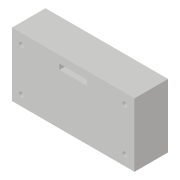
# Autodesk Inventor part: Display
Saved by Autodesk Inventor 2018 (Build 220112000, 112)
## iProperties
Created: 2019-01-22
Part Number: Display
Material: Generic
Document SubType Name: Modeling
Designer: ball
Density: 1 g/cm^3
Appearance: Default
Author: ball
Autodesk Inventor part; units mm, degrees
ref_plane "YZ Plane" through (0, 0, 0) normal (1, 0, 0) x (0, 1, 0)
ref_plane "XZ Plane" through (0, 0, 0) normal (0, 1, 0) x (-1, 0, 0)
sketch "Sketch1" plane through (0, 0, 0) normal (0, 0, 1) x (1, 0, 0)
  line L0 (-27.559, -14.2875) -> (27.559, -14.2875)
  line L1 (27.559, -14.2875) -> (27.559, 14.2875)
  line L2 (27.559, 14.2875) -> (-27.559, 14.2875)
  line L3 (-27.559, 14.2875) -> (-27.559, -14.2875)
  line L4 (-27.559, -14.2875) -> (27.559, 14.2875) construction
  line L5 (27.559, -14.2875) -> (-27.559, 14.2875) construction
  line L6 (0, 0) -> (0, 51.7616) construction
  line L7 (-6.223, 8.4963) -> (6.223, 8.4963)
  line L8 (6.223, 8.4963) -> (6.223, 10.9347)
  line L9 (6.223, 10.9347) -> (-6.223, 10.9347)
  line L10 (-6.223, 10.9347) -> (-6.223, 8.4963)
  line L11 (-6.223, 8.4963) -> (6.223, 10.9347) construction
  line L12 (6.223, 8.4963) -> (-6.223, 10.9347) construction
  circle A0 centre (-23.241, 9.7155) radius 1.0795
  circle A1 centre (23.241, 9.7155) radius 1.0795
  circle A2 centre (-23.241, -9.7155) radius 1.0795
  circle A3 centre (23.241, -9.7155) radius 1.0795
  point P0 (0, 9.7155)
  dimension "d0" = 55.118
  dimension "d1" = 28.575
  dimension "d2" = 12.446
  dimension "d3" = 2.4384
  dimension "d11" = 4.572
  dimension "d12" = 2.159
  dimension "d13" = 2.159
  dimension "d14" = 4.318
  dimension "d15" = 4.318
  dimension "d16" = 2.159
  dimension "d17" = 4.572
  dimension "d18" = 2.159
  constraints: 26 end point, 4 centre point, 4 midpoint, 4 parallel, 2 horizontal, 2 perpendicular, 1 point on line, 1 vertical
  measures "d0" distance of L1.end L2.end
  measures "d1" distance of L0.end L1.end
  measures "d2" distance of L8.end L9.end
  measures "d3" distance of L9.end L7.start
  measures "d11" distance from line of L2 point (0, 9.715)
  measures "d12" diameter of A0
  measures "d13" diameter of A1
  measures "d14" distance from line of L3 A0.centre
  measures "d15" distance from line of L1 A1.centre
  measures "d16" diameter of A2
  measures "d17" distance from line of L0 A2.centre
  measures "d18" diameter of A3
ref_plane "Work Plane1" through (0, 0, 11.938) normal (0, 0, 1) x (1, 0, 0)
sketch "Sketch2" plane through (0, 0, 11.938) normal (0, 0, 1) x (1, 0, 0)
  line L0 (-25.019, -11.7475) -> (25.019, -11.7475)
  line L1 (25.019, -11.7475) -> (25.019, 11.7475)
  line L2 (25.019, 11.7475) -> (-25.019, 11.7475)
  line L3 (-25.019, 11.7475) -> (-25.019, -11.7475)
  line L4 (-25.019, -11.7475) -> (25.019, 11.7475) construction
  line L5 (25.019, -11.7475) -> (-25.019, 11.7475) construction
  line L6 (27.559, 14.2875) -> (-27.559, 14.2875) projected
  line L7 (-27.559, 14.2875) -> (-27.559, -14.2875) projected
  point P0 (0, 0)
  dimension "d7" = 2.54
  dimension "d8" = 2.54
  constraints: 12 end point, 2 midpoint, 2 parallel, 1 horizontal, 1 perpendicular
  measures "d7" distance between parallel lines of L6 L2
  measures "d8" distance between parallel lines of L7 L3
extrude "Extrusion3" add sketch "Sketch1" along normal blind 15.113
ref_plane "Work Plane2" through (0, 0, 2.54) normal (0, 0, 1) x (1, 0, 0)
extrude "Extrusion6" cut sketch "Sketch2" against normal blind 12.573
sketch "Sketch4" plane through (0, 0, 11.938) normal (0, 0, -1) x (-1, 0, 0)
  circle A0 centre (-23.241, 9.7155) radius 1.0795 projected
  circle A1 centre (-23.241, 9.7155) radius 1.0795
  circle A2 centre (-23.241, 9.7155) radius 1.778
  line L0 (-25.019, -11.7475) -> (-25.019, 11.7475) projected
  circle A3 centre (23.241, 9.7155) radius 1.0795 projected
  circle A4 centre (23.241, 9.7155) radius 1.0795
  circle A5 centre (23.241, 9.7155) radius 1.778
  line L1 (25.019, 11.7475) -> (25.019, -11.7475) projected
  circle A6 centre (23.241, -9.7155) radius 1.0795 projected
  circle A7 centre (23.241, -9.7155) radius 1.0795
  circle A8 centre (23.241, -9.7155) radius 1.778
  circle A9 centre (-23.241, -9.7155) radius 1.0795 projected
  circle A10 centre (-23.241, -9.7155) radius 1.0795
  circle A11 centre (-23.241, -9.7155) radius 1.778
  point P0 (0, 0)
  constraints: 8 centre point, 8 coincident, 2 tangent
extrude "Extrusion7" add sketch "Sketch4" along normal blind 3.175
body "Solid2"
